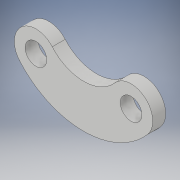
# Autodesk Inventor part: linkageC
Saved by Autodesk Inventor 2017 (Build 210142000, 142)
## iProperties
Created: 2016-08-20
Part Number: linkageC
Material: Generic
Document SubType Name: Modeling
Designer: Nic
Density: 1 g/cm^3
Appearance: Default
Author: Nic
Autodesk Inventor part; units mm, degrees
ref_plane "YZ Plane" through (0, 0, 0) normal (1, 0, 0) x (0, 1, 0)
ref_plane "XZ Plane" through (0, 0, 0) normal (0, 1, 0) x (-1, 0, 0)
ref_plane "XY Plane" through (0, 0, 0) normal (0, 0, 1) x (1, 0, 0)
sketch "Sketch1" plane through (0, 0, 0) normal (0, 0, 1) x (1, 0, 0)
  circle A0 centre (0, 0) radius 1.25
  line L0 (0, 0) -> (11, 0) construction
  circle A1 centre (11, 0) radius 1.25
  arc A2 (1.8836, 1.6438) -> (-1.8836, -1.6438) centre (0, 0) ccw
  arc A3 (12.8836, -1.6438) -> (9.1164, 1.6438) centre (11, 0) ccw
  arc A4 (-1.8836, -1.6438) -> (12.8836, -1.6438) centre (5.5, 4.8) ccw
  arc A5 (1.8836, 1.6438) -> (5.5, 0) centre (5.5, 4.8) ccw
  arc A6 (5.5, 0) -> (9.1164, 1.6438) centre (5.5, 4.8) ccw
  dimension "d0" = 2.5
  dimension "d1" = 11
  dimension "d8" = 5
  constraints: 10 point on circle, 7 centre point, 5 coincident, 5 tangent, 3 equal radius, 2 end point, 1 concentric, 1 horizontal, 1 midpoint
  measures "d0" diameter of A0
  measures "d1" distance of L0.start L0.end
  measures "d8" diameter of A2
extrude "Extrusion1" add sketch "Sketch1" along normal blind 1.5
body "Solid1"
